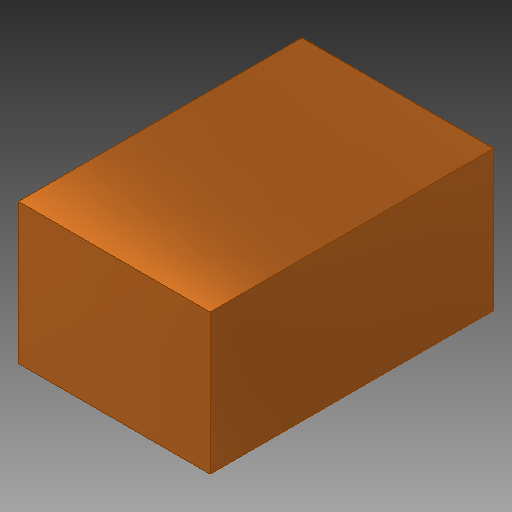
# Autodesk Inventor part: PZT
Saved by Autodesk Inventor 2017 SP1 (Build 210196100, 196)
## iProperties
Created: 2015-08-04
Part Number: PZT
Material: Gold
Document SubType Name: Modeling
Designer: Conor Mow-Lowry
Density: 19.3 g/cm^3
Appearance: Metal 1600F Hot
Author: Conor Mow-Lowry
Autodesk Inventor part; units mm, degrees
ref_plane "YZ Plane" through (0, 0, 0) normal (1, 0, 0) x (0, 1, 0)
ref_plane "XZ Plane" through (0, 0, 0) normal (0, 1, 0) x (-1, 0, 0)
ref_plane "XY Plane" through (0, 0, 0) normal (0, 0, 1) x (1, 0, 0)
sketch "Sketch1" plane through (0, 0, 0) normal (0, 0, 1) x (1, 0, 0)
  line L0 (-3.55, -2.6) -> (3.55, -2.6)
  line L1 (3.55, -2.6) -> (3.55, 2.6)
  line L2 (3.55, 2.6) -> (-3.55, 2.6)
  line L3 (-3.55, 2.6) -> (-3.55, -2.6)
  line L4 (-3.55, -2.6) -> (3.55, 2.6) construction
  line L5 (3.55, -2.6) -> (-3.55, 2.6) construction
  point P0 (0, 0)
  dimension "d0" = 7.1
  dimension "d1" = 5.2
  constraints: 12 end point, 2 midpoint, 2 parallel, 1 horizontal, 1 perpendicular
  measures "d0" distance of L1.end L2.end
  measures "d1" distance of L0.end L1.end
extrude "Extrusion1" add sketch "Sketch1" along normal blind 10.5
body "Solid1"
